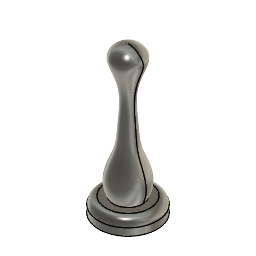
Wax Stamp Handle (Autodesk Fusion 360 design; units mm, degrees)
part number: 2026-04-06-15-47-24-760
Autodesk Fusion 360 part; units mm, degrees
sketch "Sketch1" plane through (0, 0, 0) normal (0, 1, 0) x (1, 0, 0)
  line L0 (0, 0) -> (20, 0)
  line L1 (0, 0) -> (0, -10)
  line L2 (0, -10) -> (10, -10)
  line L3 (20, 0) -> (20, -10)
  line L4 (20, -10) -> (10, -10)
  line L5 (0, 0) -> (0, -100)
  spline S0 degree 5 poles (10, -10) (10.2423, -10.4599) (10.6965, -11.3804) (11.2867, -12.7638) (11.8912, -14.6135) (12.3441, -16.9331) (12.5008, -19.2564) (12.3762, -21.5764) (11.9974, -23.8806) (11.404, -26.1537) (10.6462, -28.3849) (9.7834, -30.5727) (8.8832, -32.7324) (8.0181, -34.8984) (7.2526, -37.1153) (6.6324, -39.4306) (6.1737, -41.8869) (5.8489, -44.514) (5.6041, -47.3287) (5.3793, -50.337) (5.1282, -53.5351) (4.8359, -56.9102) (4.5443, -60.4422) (4.3447, -64.1034) (4.3447, -67.857) (4.6431, -71.6558) (5.3019, -75.4413) (6.3185, -79.1421) (7.5995, -82.6726) (8.9263, -85.9305) (10.0137, -88.8223) (10.5838, -91.2994) (10.4309, -93.3779) (9.4974, -95.1939) (7.9352, -96.9885) (5.8174, -98.6062) (3.7253, -99.5443) (1.9441, -99.9171) (0.6636, -100) (0, -100) knots 0 0 0 0 0 0 0.028571 0.057143 0.085714 0.114286 0.142857 0.171429 0.2 0.228571 0.257143 0.285714 0.314286 0.342857 0.371429 0.4 0.428571 0.457143 0.485714 0.514286 0.542857 0.571429 0.6 0.628571 0.657143 0.685714 0.714286 0.742857 0.771429 0.8 0.828571 0.857143 0.885714 0.914286 0.942857 0.971429 1 1 1 1 1 1
  line L6 (12.5504, -87.9691) -> (7.4496, -100.0208)
  line L7 (11.5931, -100) -> (-11.5931, -100)
  point P0 (12.4144, -20.2134)
  point P1 (10, -30)
  point P2 (6.6101, -39.7471)
  point P3 (5, -55)
  point P4 (6.5317, -79.562)
  point P5 (10, -93.995)
  dimension "d1" = 20
  constraint coincident L0.start L1.start
  constraint horizontal L0
  constraint perpendicular L1 L2
  constraint perpendicular L0 L3
  constraint perpendicular L3 L4
  constraint perpendicular L0 L5
  constraint midpoint P5 L6
  constraint midpoint L5.end L7
  measures "d1" distance of L0.start L0.end
revolve "Revolve1" add sketch "Sketch1" angle 360 about axis through (0, 0, 1.75) along (0, 0, 1) contours L0 L1 L2 L3 L4 L5 | L2 L5 S0
fillet "Fillet1" radius 5 1 edges at (-18.6465, -7.2323, 10)
